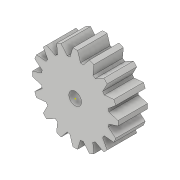
# Autodesk Inventor part: g
Saved by Autodesk Inventor 2019 (Build 230136000, 136)
## iProperties
Created: 2023-07-28
Part Number: g
Material: Generic
Document SubType Name: Modeling
Designer: ahmed
Density: 1 g/cm^3
Appearance: Default
Author: ahmed
## iProperties of the stored document g_3DPrint.ipt
Created: 2023-07-29
Part Number: g_3DPrint
Material: Generic
Document SubType Name: Modeling
Designer: ahmed
Density: 1 g/cm^3
Appearance: Default
Author: ahmed
Autodesk Inventor part; units mm, degrees
ref_plane "YZ Plane" through (0, 0, 0) normal (1, 0, 0) x (0, 1, 0)
ref_plane "XZ Plane" through (0, 0, 0) normal (0, 1, 0) x (-1, 0, 0)
ref_plane "XY Plane" through (0, 0, 0) normal (0, 0, 1) x (1, 0, 0)
sketch "Sketch1" plane through (0, 0, 0) normal (0, 0, 1) x (1, 0, 0)
  circle A0 centre (0, 0) radius 2.15
  arc A1 (0.799, 14.478) -> (-0.799, 14.478) centre (0, 0) ccw
  line L0 (-0.799, 14.478) -> (-1.7026, 11.4992)
  line L1 (-1.7026, 11.4992) -> (-1.7434, 11.3646)
  line L2 (0.799, 14.478) -> (1.9203, 10.9587)
  line L3 (1.7935, 11.3568) -> (1.9203, 10.9587)
  arc A2 (-4.8023, 13.6817) -> (-6.2787, 13.0701) centre (0, 0) ccw
  line L4 (-6.2787, 13.0701) -> (-5.9735, 9.9724)
  line L5 (-5.9735, 9.9724) -> (-5.9597, 9.8323)
  line L6 (-4.8023, 13.6817) -> (-2.4196, 10.8594)
  line L7 (-2.6891, 11.1786) -> (-2.4196, 10.8594)
  arc A3 (-9.6725, 10.8025) -> (-10.8025, 9.6725) centre (0, 0) ccw
  line L8 (-10.8025, 9.6725) -> (-9.3351, 6.9273)
  line L9 (-9.3351, 6.9273) -> (-9.2687, 6.8032)
  line L10 (-9.6725, 10.8025) -> (-6.3911, 9.1068)
  line L11 (-6.7623, 9.2986) -> (-6.3911, 9.1068)
  arc A4 (-13.0701, 6.2787) -> (-13.6817, 4.8023) centre (0, 0) ccw
  line L12 (-13.6817, 4.8023) -> (-11.2755, 2.8276)
  line L13 (-11.2755, 2.8276) -> (-11.1667, 2.7384)
  line L14 (-13.0701, 6.2787) -> (-9.3896, 5.9678)
  line L15 (-9.806, 6.003) -> (-9.3896, 5.9678)
  arc A5 (-14.478, 0.799) -> (-14.478, -0.799) centre (0, 0) ccw
  line L16 (-14.478, -0.799) -> (-11.4992, -1.7026)
  line L17 (-11.4992, -1.7026) -> (-11.3646, -1.7434)
  line L18 (-14.478, 0.799) -> (-10.9587, 1.9203)
  line L19 (-11.3568, 1.7935) -> (-10.9587, 1.9203)
  arc A6 (-13.6817, -4.8023) -> (-13.0701, -6.2787) centre (0, 0) ccw
  line L20 (-13.0701, -6.2787) -> (-9.9724, -5.9735)
  line L21 (-9.9724, -5.9735) -> (-9.8323, -5.9597)
  line L22 (-13.6817, -4.8023) -> (-10.8594, -2.4196)
  line L23 (-11.1786, -2.6891) -> (-10.8594, -2.4196)
  arc A7 (-10.8025, -9.6725) -> (-9.6725, -10.8025) centre (0, 0) ccw
  line L24 (-9.6725, -10.8025) -> (-6.9273, -9.3351)
  line L25 (-6.9273, -9.3351) -> (-6.8032, -9.2687)
  line L26 (-10.8025, -9.6725) -> (-9.1068, -6.3911)
  line L27 (-9.2986, -6.7623) -> (-9.1068, -6.3911)
  arc A8 (-6.2787, -13.0701) -> (-4.8023, -13.6817) centre (0, 0) ccw
  line L28 (-4.8023, -13.6817) -> (-2.8276, -11.2755)
  line L29 (-2.8276, -11.2755) -> (-2.7384, -11.1667)
  line L30 (-6.2787, -13.0701) -> (-5.9678, -9.3896)
  line L31 (-6.003, -9.806) -> (-5.9678, -9.3896)
  arc A9 (-0.799, -14.478) -> (0.799, -14.478) centre (0, 0) ccw
  line L32 (0.799, -14.478) -> (1.7026, -11.4992)
  line L33 (1.7026, -11.4992) -> (1.7434, -11.3646)
  line L34 (-0.799, -14.478) -> (-1.9203, -10.9587)
  line L35 (-1.7935, -11.3568) -> (-1.9203, -10.9587)
  arc A10 (4.8023, -13.6817) -> (6.2787, -13.0701) centre (0, 0) ccw
  line L36 (6.2787, -13.0701) -> (5.9735, -9.9724)
  line L37 (5.9735, -9.9724) -> (5.9597, -9.8323)
  line L38 (4.8023, -13.6817) -> (2.4196, -10.8594)
  line L39 (2.6891, -11.1786) -> (2.4196, -10.8594)
  arc A11 (9.6725, -10.8025) -> (10.8025, -9.6725) centre (0, 0) ccw
  line L40 (10.8025, -9.6725) -> (9.3351, -6.9273)
  line L41 (9.3351, -6.9273) -> (9.2687, -6.8032)
  line L42 (9.6725, -10.8025) -> (6.3911, -9.1068)
  line L43 (6.7623, -9.2986) -> (6.3911, -9.1068)
  arc A12 (13.0701, -6.2787) -> (13.6817, -4.8023) centre (0, 0) ccw
  line L44 (13.6817, -4.8023) -> (11.2755, -2.8276)
  line L45 (11.2755, -2.8276) -> (11.1667, -2.7384)
  line L46 (13.0701, -6.2787) -> (9.3896, -5.9678)
  line L47 (9.806, -6.003) -> (9.3896, -5.9678)
  arc A13 (14.478, -0.799) -> (14.478, 0.799) centre (0, 0) ccw
  line L48 (14.478, 0.799) -> (11.4992, 1.7026)
  line L49 (11.4992, 1.7026) -> (11.3646, 1.7434)
  line L50 (14.478, -0.799) -> (10.9587, -1.9203)
  line L51 (11.3568, -1.7935) -> (10.9587, -1.9203)
  arc A14 (13.6817, 4.8023) -> (13.0701, 6.2787) centre (0, 0) ccw
  line L52 (13.0701, 6.2787) -> (9.9724, 5.9735)
  line L53 (9.9724, 5.9735) -> (9.8323, 5.9597)
  line L54 (13.6817, 4.8023) -> (10.8594, 2.4196)
  line L55 (11.1786, 2.6891) -> (10.8594, 2.4196)
  arc A15 (10.8025, 9.6725) -> (9.6725, 10.8025) centre (0, 0) ccw
  line L56 (9.6725, 10.8025) -> (6.9273, 9.3351)
  line L57 (6.9273, 9.3351) -> (6.8032, 9.2687)
  line L58 (10.8025, 9.6725) -> (9.1068, 6.3911)
  line L59 (9.2986, 6.7623) -> (9.1068, 6.3911)
  arc A16 (6.2787, 13.0701) -> (4.8023, 13.6817) centre (0, 0) ccw
  line L60 (4.8023, 13.6817) -> (2.8276, 11.2755)
  line L61 (2.8276, 11.2755) -> (2.7384, 11.1667)
  line L62 (6.2787, 13.0701) -> (5.9678, 9.3896)
  line L63 (6.003, 9.806) -> (5.9678, 9.3896)
  arc A17 (-1.7434, 11.3646) -> (-2.6891, 11.1786) centre (0, 0) ccw
  arc A18 (-5.9597, 9.8323) -> (-6.7623, 9.2986) centre (0, 0) ccw
  arc A19 (-9.2687, 6.8032) -> (-9.806, 6.003) centre (0, 0) ccw
  arc A20 (-11.1667, 2.7384) -> (-11.3568, 1.7935) centre (0, 0) ccw
  arc A21 (-11.3646, -1.7434) -> (-11.1786, -2.6891) centre (0, 0) ccw
  arc A22 (-9.8323, -5.9597) -> (-9.2986, -6.7623) centre (0, 0) ccw
  arc A23 (-6.8032, -9.2687) -> (-6.003, -9.806) centre (0, 0) ccw
  arc A24 (-2.7384, -11.1667) -> (-1.7935, -11.3568) centre (0, 0) ccw
  arc A25 (1.7434, -11.3646) -> (2.6891, -11.1786) centre (0, 0) ccw
  arc A26 (5.9597, -9.8323) -> (6.7623, -9.2986) centre (0, 0) ccw
  arc A27 (9.2687, -6.8032) -> (9.806, -6.003) centre (0, 0) ccw
  arc A28 (11.1667, -2.7384) -> (11.3568, -1.7935) centre (0, 0) ccw
  arc A29 (11.3646, 1.7434) -> (11.1786, 2.6891) centre (0, 0) ccw
  arc A30 (9.8323, 5.9597) -> (9.2986, 6.7623) centre (0, 0) ccw
  arc A31 (6.8032, 9.2687) -> (6.003, 9.806) centre (0, 0) ccw
  arc A32 (2.7384, 11.1667) -> (1.7935, 11.3568) centre (0, 0) ccw
  dimension "d0" = 4.3
  dimension "d1" = 29
  dimension "d11" = 360
  constraints: 128 end point, 64 point on circle, 33 centre point, 16 point on line, 2 coincident, 1 collinear, 193 other
  measures "d0" diameter of A0
  measures "d1" diameter of A1
extrude "Extrusion1" add sketch "Sketch1" along normal blind 10
sketch "Sketch2" plane through (0, 0, 10) normal (0, 0, 1) x (1, 0, 0)
  point P0 (0, 0)
body "Solid1"
